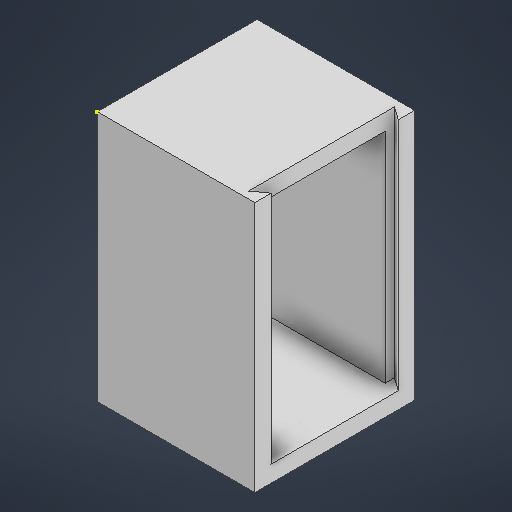
# Autodesk Inventor part: Part4
Saved by Autodesk Inventor 2026.1 (Build 301233000, 233)
## iProperties
Created: 2025-08-22
Part Number: Part4
Material: Generic
Document SubType Name: Modeling
Designer: usman
Density: 1 g/cm^3
Appearance: Default
Author: usman
Autodesk Inventor part; units mm, degrees
ref_plane "YZ Plane" through (0, 0, 0) normal (1, 0, 0) x (0, 1, 0)
ref_plane "XZ Plane" through (0, 0, 0) normal (0, 1, 0) x (-1, 0, 0)
ref_plane "XY Plane" through (0, 0, 0) normal (0, 0, 1) x (1, 0, 0)
sketch "Sketch1" plane through (0, 0, 0) normal (1, 0, 0) x (0, 1, 0)
  line L0 (0, 0) -> (191.4, 0)
  line L1 (191.4, 0) -> (191.4, -121.8)
  line L2 (191.4, -121.8) -> (0, -121.8)
  line L3 (0, -121.8) -> (0, 0)
  dimension "d0" = 191.4
  dimension "d1" = 121.8
  constraints: 8 end point, 2 parallel, 1 horizontal, 1 perpendicular
  measures "d0" distance of L0.start L0.end
  measures "d1" distance of L0.end L1.end
extrude "Extrusion1" add sketch "Sketch1" along normal blind 120
sketch "Sketch2" plane through (120, 0, 0) normal (1, 0, 0) x (0, 0, -1)
  line L0 (12.4, 178.9) -> (109.4, 178.9)
  line L1 (109.4, 178.9) -> (109.4, 12.5)
  line L2 (109.4, 12.5) -> (12.4, 12.5)
  line L3 (12.4, 12.5) -> (12.4, 178.9)
  line L4 (121.8, 191.4) -> (0, 191.4) projected
  line L5 (0, 0) -> (121.8, 0) projected
  line L6 (0, 191.4) -> (0, 0) projected
  dimension "d4" = 12.5
  dimension "d5" = 12.5
  dimension "d6" = 12.4
  dimension "d7" = 97
  constraints: 8 end point, 2 parallel, 1 horizontal, 1 perpendicular
  measures "d4" distance between parallel lines of L4 L0
  measures "d5" distance between parallel lines of L5 L2
  measures "d6" distance between parallel lines of L6 L3
  measures "d7" distance of L1.end L2.end
extrude "Extrusion2" cut sketch "Sketch2" against normal blind 105
sketch "Sketch3" plane through (0, 191.4, 0) normal (0, 1, 0) x (1, 0, 0)
  point P0 (0, 0)
sketch "Sketch4" plane through (0, 191.4, 0) normal (0, 1, 0) x (1, 0, 0)
  line L0 (120, 109.4) -> (15, 109.4) projected
  line L1 (120, 109.4) -> (110, 116.4021)
  line L2 (120, 121.8) -> (120, 0) projected
  line L3 (120, 60.9) -> (110, 60.9)
  line L4 (110, 60.9) -> (110, 116.4021)
  line L5 (120, 109.4) -> (120, 60.9)
  point P0 (0, 0)
  point P1 (106.1473, 60.9)
  dimension "d10" = 55
  dimension "d11" = 10
  constraints: 8 end point, 1 collinear, 1 horizontal, 1 midpoint, 1 perpendicular
  measures "d10" angle of L2 L1
  measures "d11" horizontal distance of L0.start L1.end
extrude "Extrusion3" cut sketch "Sketch4" against normal up to surface (178.9 mm away)
sketch "Sketch5" plane through (0, 191.4, 0) normal (0, 1, 0) x (1, 0, 0)
  line L0 (120, 109.4) -> (120, 12.4) projected
  line L1 (120, 12.4) -> (15, 12.4) projected
  line L2 (120, 60.9) -> (120, 12.4)
  line L3 (120, 12.4) -> (110, 5.3979)
  line L4 (120, 60.9) -> (120, 0) projected
  line L5 (110, 109.4) -> (110, 60.9) projected
  line L6 (110, 60.9) -> (110, 5.3979)
  line L7 (110, 60.9) -> (110, 5.3979)
  line L8 (110, 60.9) -> (120, 60.9) projected
  line L9 (120, 60.9) -> (110, 60.9)
  point P0 (0, 0)
  dimension "d14" = 10
  dimension "d15" = 125
  constraints: 10 end point, 2 collinear, 1 midpoint, 1 perpendicular, 1 vertical
  measures "d14" horizontal distance of L0.end L3.end
  measures "d15" angle of L4 L3
extrude "Extrusion4" cut sketch "Sketch5" against normal up to surface (178.9 mm away)
body "Solid1"
